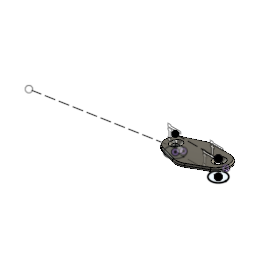
mirror blank v5 (Autodesk Fusion 360 design; units mm, degrees)
Autodesk Fusion 360 part; units mm, degrees
sketch "Sketch1" plane through (0, 0, 0) normal (0, 0, 1) x (1, 0, 0)
  line L0 (0, 0) -> (43.7, 0) construction
  circle A0 centre (0, 0) radius 8.2
  circle A1 centre (43.7, 0) radius 7.5
  dimension "d1" = 43.7
  dimension "d2" = 16.4
  dimension "d3" = 15
  constraint coincident L0.start A0.centre
  constraint horizontal L0
  constraint coincident L0.end A1.centre
  measures "d1" distance of L0.start L0.end
  measures "d2" diameter of A0
  measures "d3" diameter of A1
extrude "Extrude1" add sketch "Sketch1" along normal blind 5 contours A0 makes body 1
extrude "Extrude2" add sketch "Sketch1" along normal blind 4.4 from surface at 7.2 separate body contours A1 makes body 2
sketch "Sketch2" plane through (0, 0, 11.6) normal (0, 0, 1) x (-1, 0, 0)
  circle A0 centre (-43.7, 0) radius 7.5
  line L0 (-51.2, 20) -> (-51.2, -20) construction
  point P0 (-51.2, 0)
  constraint vertical L0
  constraint tangent A0 L0
  constraint midpoint L0 P0
sketch "Sketch3" plane through (0, 0, 5) normal (0, 0, 1) x (-1, 0, 0)
  circle A0 centre (0, 0) radius 8.2
  line L0 (-8.2, 20) -> (-8.2, -20) construction
  point P0 (-8.2, 0)
  constraint vertical L0
  constraint tangent A0 L0
  constraint midpoint L0 P0
sketch "Sketch4" plane through (0, 0, 0) normal (0, 1, 0) x (1, 0, 0)
  line L0 (4.7376, -4.4686) -> (-148.7072, 19.0834) construction
  line L1 (43.7, 0) -> (43.7, -16) construction
  line L2 (0, 0) -> (0, -16) construction
  line L3 (0, -16) -> (43.7, -16) construction
  point P0 (8.2, -5)
  point P1 (51.2, -11.6)
  point P2 (43.7, 0)
  point P3 (0, -16)
  point P4 (43.7, -16)
  dimension "d27" = 16
  dimension "d28" = 16
  constraint coincident L0 P0
  constraint coincident L0 P1
  constraint coincident P2 L1.start
  constraint coincident L2.start origin
  constraint perpendicular L1 L3
  constraint vertical L2
  constraint coincident P3 L2.end
  constraint coincident P4 L1.end
  measures "d27" distance of L2.start P3
  measures "d28" distance of P2 P4
ref_plane "WorkPlane1" through (-71.9848, 0, -7.3074) normal (-0.151712, 0, 0.988425) x (-0.988425, 0, -0.151712)
sketch "Sketch5" plane through (6.6692, 0, 4.765) normal (-0.151712, 0, 0.988425) x (-0.988425, 0, -0.151712)
  line L0 (-37.6379, 0, 1.13) -> (6.5738, 0, 1.13)
  line L1 (-35.8793, 0, -10.3279) -> (-38.3067, 0, 5.4869)
  line L2 (7.3149, 0, -3.6981) -> (4.8875, 0, 12.1167)
  circle A0 through (0.318, 0, 1.13) (-23.457, 13.7265, 1.13) (-23.457, -13.7265, 1.13)
  circle A1 through (17.2738, 0, 1.13) (1.2238, 9.2665, 1.13) (1.2238, -9.2665, 1.13)
  circle A2 through (-25.6379, 0, 1.13) (-43.6379, 10.3923, 1.13) (-43.6379, -10.3923, 1.13)
  line L3 (10.5187, 9.9463, 1.13) -> (-8.5824, 17.5221, 1.13)
  line L4 (-21.3731, 17.9222, 1.13) -> (-41.3564, 11.4093, 1.13)
  line L5 (-39.7279, -11.8166, 1.13) -> (-18.2925, -15.6078, 1.13)
  line L6 (-11.8395, -15.4139, 1.13) -> (9.0666, -10.4056, 1.13)
  circle A3 through (3.318, 0, 1.13) (-24.957, 16.3246, 1.13) (-24.957, -16.3246, 1.13)
  point P0 (-15.532, 0)
  dimension "d13" = 31.7
  dimension "d17" = 21.4
  dimension "d18" = 24
  dimension "d45" = 37.7
extrude "Extrude3" add sketch "Sketch5" along normal blind 1.5 contours L0 A0 A1 A3 | L0 A0 A1 | L0 A0 A1 | L0 A0 A1 A3 | A1 A3 | L0 A0 A1 A2 | L0 A0 A1 A2 | A0 A1 A2 A3 | A0 A1 L6 A3 | A1 L3 A3 | A1 L6 A3 | L0 A0 A2 | L0 A0 A2 | L0 A0 A2 A3 | L0 A0 A2 A3 | A0 A2 L5 A3 | A2 A3 | A2 L4 A3 | A2 L5 A3 in plane through (6.4977, 0, 5.882) normal (-0.151712, 0, 0.988425) bodies 1 2
extrude "Extrude4" add 1 faces at (32.4283, 3.1674, 11.3796) along direction (-0.151712, 0, 0.988425) blind 1.5 draft -30 on bodies 1 bodies 1
extrude "Extrude5" add sketch "Sketch2" along normal up to surface end surface through (6.0426, 0, 8.8472) normal (-0.151712, 0, 0.988425) offset 0 bodies 1
extrude "Extrude6" add sketch "Sketch3" along normal up to surface end surface through (6.0426, 0, 8.8472) normal (-0.151712, 0, 0.988425) offset 0 bodies 1
ref_plane "WorkPlane2" through (21.85, 0, 16) normal (0, 0, 1) x (1, 0, 0)
hole "Hole1" at (0, 0, 16) direction (0, 0, -1) diameter 6 depth 30 tip angle 118 countersink diameter 27 countersink angle 90 bodies 1
sketch "Sketch6" plane through (21.85, 0, 16) normal (0, 0, 1) x (1, 0, 0)
  point P0 (21.85, 0)
  point P1 (21.85, 0)
  constraint coincident P0 P1
hole "Hole2" at (43.7, 0, 16) direction (0, 0, -1) diameter 6 depth 30 tip angle 118 countersink diameter 14 countersink angle 90 bodies 1
extrude "Extrude7" cut sketch "Sketch1" along normal blind 3 contours A0 bodies 1
extrude "Extrude8" cut 1 faces at (49.6693, -0.4473, 7.2) along direction (0, 0, 1) blind 3 on bodies 1 bodies 1
equation "d1 = 49.5 mm - 5.8 mm"
equation "d2 = bigend"
equation "d3 = smallend"
equation "firststep = 4.7 mm"
equation "secondstep = 2.5 mm"
equation "d8 = firststep + secondstep"
equation "middlewidth = 26.7 mm + overlap"
equation "d13 = middlewidth"
equation "bigend = 16.4 mm"
equation "smallend = 15 mm"
equation "overlap = 5 mm"
equation "d17 = bigend + overlap"
equation "d18 = smallend + overlap + 4 mm"
equation "bigmiddlewidth = middlewidth + 6 mm"
equation "d45 = bigmiddlewidth"
named bodies: "mirror blank"
